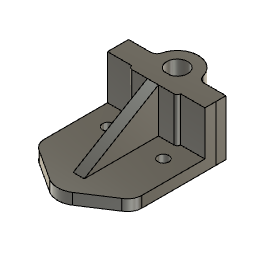
a3 (Autodesk Fusion 360 design; units mm, degrees)
Autodesk Fusion 360 part; units mm, degrees
note: some values were not read from the file. Set by a fixed rule: which sketch regions a step uses.
sketch "Sketch1" plane through (0, 0, 0) normal (0, 0, 1) x (1, 0, 0)
  line L0 (-44, 15.5) -> (44, 15.5)
  line L1 (44, 15.5) -> (44, -15.5)
  line L2 (-44, -15.5) -> (-44, 15.5)
  line L3 (-44, 15.5) -> (44, -15.5) construction
  line L4 (44, 15.5) -> (-44, -15.5) construction
  circle A0 centre (-25, 0) radius 5
  circle A1 centre (25, 0) radius 5
  line L5 (-44, -15.5) -> (-44, -38.5)
  line L6 (44, -38.5) -> (44, -15.5)
  line L7 (-44, 15.5) -> (44, 15.5)
  line L8 (44, 15.5) -> (44, 28.5)
  line L9 (44, 28.5) -> (-44, 28.5)
  line L10 (-44, 28.5) -> (-44, 15.5)
  line L11 (0, -51.5) -> (-5, -51.5)
  line L12 (0, -51.5) -> (5, -51.5)
  line L13 (-5, -51.5) -> (-5, 15.5)
  line L14 (5, -51.5) -> (5, 15.5)
  line L15 (-37.3007, -49.8711) -> (-10.3733, -67.4184)
  line L16 (37.3007, -49.8711) -> (10.3733, -67.4184)
  arc A2 (-10.3733, -67.4184) -> (10.3733, -67.4184) centre (0, -51.5) ccw
  arc A3 (37.3007, -49.8711) -> (44, -38.5) centre (31, -38.5) ccw
  arc A4 (-44, -38.5) -> (-37.3007, -49.8711) centre (-31, -38.5) ccw
  dimension "d1" = 31
  dimension "d2" = 88
  dimension "d3" = 10
  dimension "d4" = 10
  dimension "d5" = 50
  dimension "d6" = 19
  dimension "d7" = 19
  dimension "d9" = 38
  dimension "d12" = 13
  dimension "d13" = 5
  dimension "d14" = 5
  dimension "d15" = 26
  dimension "d16" = 26
  constraint perpendicular L0 L1
  constraint parallel L1 L2
  constraint horizontal L0
  constraint coincident L3 origin
  constraint coincident L4 origin
  constraint vertical L5
  constraint vertical L6
  constraint horizontal L7
  constraint vertical L8
  constraint horizontal L9
  constraint vertical L10
  constraint coincident L11.start L12.start
  constraint coincident L7 L13.end
  constraint perpendicular L7 L13
  constraint coincident L7 L14.end
  constraint perpendicular L7 L14
  constraint tangent L5 A4
  constraint tangent L6 A3
  constraint tangent L15 A2
  constraint tangent L16 A2
  measures "d1" distance of L0.end L1.end
  measures "d2" distance of L1.end L2.start
  measures "d3" diameter of A0
  measures "d4" diameter of A1
  measures "d5" distance of A0.centre A1.centre
  measures "d6" distance of L2 A0.centre
  measures "d7" distance of L1 A1.centre
  measures "d9" diameter of A2
  measures "d12" distance of L0.start L9.end
  measures "d13" distance of L11.start L11.end
  measures "d14" distance of L11.start L12.end
  measures "d15" diameter of A4
  measures "d16" diameter of A3
extrude "Extrude1" add sketch "Sketch1" along normal blind 10 contours L0 L1 L2 L5 L6 L7 L11 L12 L13 L14 L15 L16 A2 A3 A4
extrude "Extrude2" add sketch "Sketch1" along normal blind 50 contours L0 L7 L8 L9 L10
extrude "Extrude3" add sketch "Sketch1" along normal blind 50 contours L0 L7 L11 L12 L13 L14
sketch "Sketch2" plane through (0, 0, 50) normal (0, 0, 1) x (-1, 0, 0)
  line L0 (44, -28.5) -> (44, -15.5)
  line L1 (44, -15.5) -> (5, -15.5)
  line L2 (5, -15.5) -> (5, 51.5)
  line L3 (5, 51.5) -> (-5, 51.5)
  line L4 (-5, 51.5) -> (-5, -15.5)
  line L5 (-5, -15.5) -> (-44, -15.5)
  line L6 (-44, -15.5) -> (-44, -28.5)
  line L7 (-44, -28.5) -> (44, -28.5)
  circle A0 centre (19, -18.5) radius 3
  circle A1 centre (-19, -18.5) radius 3
  line L8 (19, -18.5) -> (44, -18.5)
  line L9 (-19, -18.5) -> (-44, -18.5)
  line L10 (44, -18.5) -> (44, -15.5)
  line L11 (19, -15.5) -> (19, -18.5)
  line L12 (-19, -18.5) -> (-19, -15.5)
  line L13 (-19, -18.5) -> (-19, -15.5)
  line L14 (-44, -15.5) -> (-44, -18.5)
  line L15 (44, -18.5) -> (44, -37.5)
  line L16 (44, -37.5) -> (-44, -37.5)
  line L17 (-44, -37.5) -> (-44, -18.5)
  circle A2 centre (0, -37.5) radius 9.5
  circle A3 centre (0, -37.5) radius 19
  arc A4 (24.2693, -37.5) -> (18.4447, -42.06) centre (24.2693, -43.5) ccw
  arc A5 (-18.4447, -42.06) -> (-24.2693, -37.5) centre (-24.2693, -43.5) ccw
  dimension "d23" = 6
  dimension "d24" = 6
  dimension "d25" = 38
  dimension "d26" = 25
  dimension "d31" = 19
  dimension "d32" = 19
  dimension "d33" = 38
  dimension "d35" = 12
  dimension "d36" = 12
  constraint tangent L1 A0
  constraint tangent L5 A1
  constraint coincident A0.centre L8.start
  constraint coincident L0 L8.end
  constraint perpendicular L0 L8
  constraint coincident A1.centre L9.start
  constraint coincident L6 L9.end
  constraint perpendicular L6 L9
  constraint coincident L0.end L1.start
  constraint coincident A0 L11.start
  constraint perpendicular L8 L11
  constraint coincident A1 L12.end
  constraint perpendicular L5 L12
  constraint coincident L5.end L6.start
  constraint perpendicular L7 L15
  constraint perpendicular L6 L16
  constraint parallel L14 L17
  constraint midpoint L16 A2.centre
  constraint concentric A2 A3
  constraint tangent A3 A5
  constraint tangent L16 A5
  constraint tangent A3 A4
  constraint tangent L16 A4
  constraint coincident A3 A4.end
  constraint coincident L16 A4.start
  constraint coincident L16 A5.end
  constraint coincident A3 A5.start
  measures "d23" diameter of A0
  measures "d24" diameter of A1
  measures "d25" distance of A0.centre A1.centre
  measures "d26" distance of L0 A0.centre
  measures "d31" distance of L8.end L15.end
  measures "d32" diameter of A2
  measures "d33" diameter of A3
  measures "d35" diameter of A5
  measures "d36" diameter of A4
extrude "Extrude4" cut sketch "Sketch2" against normal blind 40 contours L0 L1 A0 L8 L10
extrude "Extrude5" cut sketch "Sketch2" against normal blind 40 contours L5 L6 A1 L9 L14
sketch "Sketch3" plane through (0, 0, 50) normal (0, 0, 1) x (-1, 0, 0)
extrude "Extrude6" add sketch "Sketch2" against normal blind 50 contours L7 L15 L16 A3 | L7 L16 A2 A3 | L16 A2 A3 | L16 A3 A4 | L7 L16 L17 A3 | L7 L16 A2 A3 | L16 A3 A5
sketch "Sketch4" plane through (-5, 0, 0) normal (-1, 0, 0) x (0, -1, 0)
  line L0 (-15.5, 10) -> (51.5, 10)
  line L1 (51.5, 10) -> (51.5, 50)
  line L2 (51.5, 50) -> (-15.5, 50)
  line L3 (-15.5, 50) -> (-15.5, 10)
  line L4 (-15.5, 50) -> (51.5, 10)
  constraint coincident L2.end L3.start
  constraint coincident L0.end L1.start
extrude "Extrude7" cut sketch "Sketch4" against normal blind 85 contours L1 L2 L4
equation "d6 = ( ( 88 - 50 ) / 2 ) * 1 mm"
equation "d9 = ( 19 * 2 ) * 1 mm"
equation "d26 = ( ( 88 - 38 ) / 2 ) * 1 mm"
equation "d33 = ( 19 * 2 ) * 1 mm"
